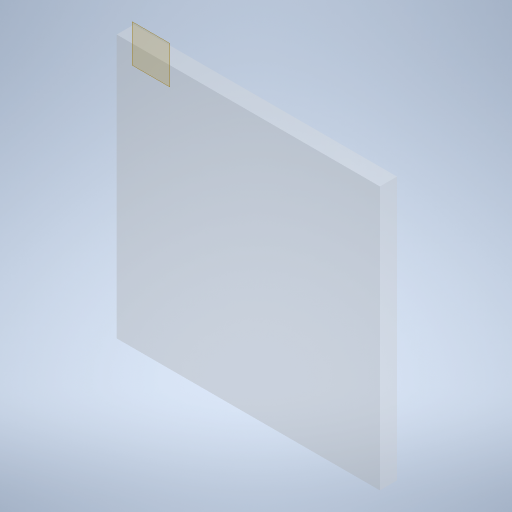
# Autodesk Inventor part: Acrylic
Saved by Autodesk Inventor 2023 (Build 270158000, 158)
## iProperties
Created: 2025-01-02
Part Number: Acrylic
Material: Generic
Document SubType Name: Modeling
Designer: jonwo
Density: 1 g/cm^3
Appearance: Polycarbonate - Clear
Author: jonwo
Autodesk Inventor part; units mm, degrees
ref_plane "YZ Plane" through (0, 0, 0) normal (1, 0, 0) x (0, 1, 0)
ref_plane "XZ Plane" through (0, 0, 0) normal (0, 1, 0) x (-1, 0, 0)
ref_plane "XY Plane" through (0, 0, 0) normal (0, 0, 1) x (1, 0, 0)
ref_plane "Work Plane1" through (0, 0, 0) normal (0, 0, 1) x (1, 0, 0)
sketch "Sketch1" plane through (0, 0, 0) normal (0, 0, 1) x (1, 0, 0)
  line L0 (7.366, 7.366) -> (7.366, 56.134) projected
  line L1 (7.366, 56.134) -> (56.134, 56.134) projected
  line L2 (56.134, 56.134) -> (56.134, 7.366) projected
  line L3 (56.134, 7.366) -> (7.366, 7.366) projected
  point P0 (0, 0)
extrude "Extrusion1" add sketch "Sketch1" along normal blind 3.175
equation "\"d13\" = acrylicthickness"
equation "\"d0\" = 63.5"
equation "\"d1\" = 63.5"
equation "\"d2\" = 63.5"
equation "\"d3\" = 0"
equation "\"d4\" = 7.366"
equation "\"d5\" = 79.6925"
equation "\"d6\" = 0"
equation "\"outerprofile\" = 63.5"
equation "\"innerprofile\" = 48.768"
equation "\"overalldepth\" = 63.5"
equation "\"wirechannelwidth\" = 8"
equation "\"wirechanneldepth\" = 3"
equation "\"frontpanelsupports\" = 6.35"
equation "\"outerfillets\" = 7.366"
equation "\"supportfillets\" = 6.35"
equation "\"d7\" = outerprofile"
equation "\"d8\" = outerprofile"
equation "\"d9\" = overalldepth"
equation "\"d10\" = 0"
equation "\"acrylicthickness\" = 3.175"
equation "\"trimwidth\" = 25.4"
equation "\"trimdepth\" = 5.08"
equation "\"d11\" = innerprofile"
equation "\"d14\" = 0"
equation "\"patternspacing\" = innerprofile - frontpanelsupports"
equation "\"wirechannelspacing\" = 10.795"
equation "\"controllerseatbeltheight\" = 10.16"
equation "\"controllerseatbeltwidth\" = 15.24"
equation "\"wirechannelfillets\" = 25.4"
equation "\"d41\" = outerfillets"
equation "\"d42\" = outerfillets"
equation "\"d44\" = 1.6"
equation "\"d45\" = controllerseatbeltheight"
equation "\"d55\" = 1.6"
equation "\"d56\" = controllerseatbeltheight"
equation "\"d57\" = controllerseatbeltwidth"
equation "\"d58\" = 2 * supportfillets"
equation "\"d59\" = 19.05"
equation "\"d60\" = 0"
equation "\"d61\" = supportfillets"
equation "\"d62\" = supportfillets"
equation "\"d63\" = 0"
equation "\"d64\" = 0"
equation "\"d65\" = 0.372"
equation "\"d79\" = 2.9972"
equation "\"pcblength\" = 32"
equation "\"d103\" = 1.35"
equation "\"d104\" = 18.25"
equation "\"d108\" = 4.6"
equation "\"d111\" = d108"
equation "\"d112\" = 1.2"
equation "\"d113\" = 0"
equation "\"d114\" = 3.6"
equation "\"d115\" = 4.6"
equation "\"d116\" = 4.6"
equation "\"d117\" = 6.5"
equation "\"d118\" = 0"
equation "\"d119\" = 1.4"
equation "\"d120\" = 15"
equation "\"d121\" = 0"
equation "\"d122\" = 0.5"
equation "\"d123\" = 3.8"
equation "\"d124\" = 4.75"
equation "\"d125\" = d124"
equation "\"d127\" = 2.4"
equation "\"d129\" = 0"
equation "\"d132\" = 3"
equation "\"d133\" = wirechannelwidth"
equation "\"d135\" = wirechannelwidth"
equation "\"d136\" = 2"
equation "\"d141\" = wirechanneldepth"
equation "\"d142\" = 0"
equation "\"d143\" = wirechanneldepth"
equation "\"d152\" = 0.5"
equation "\"d153\" = 0.9"
equation "\"d154\" = 0.8"
equation "\"d155\" = 0"
equation "\"wing\" = 6.25"
equation "\"d157\" = 2 * wirechanneldepth"
equation "\"d158\" = 2"
equation "\"d160\" = wing"
equation "\"d161\" = wing"
equation "\"d162\" = 3"
equation "\"d165\" = 0"
equation "\"d166\" = 2"
equation "\"d167\" = 0.5"
equation "\"d168\" = 4"
equation "\"d172\" = -0.7"
equation "\"ledsandwich\" = 2 * acrylicthickness + ledwidth + trimdepth"
equation "\"d12\" = -ledsandwich"
equation "\"d126\" = d127"
equation "\"ledwidth\" = 10"
body "Solid1"
